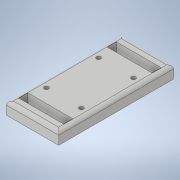
# Autodesk Inventor part: Tilt_Camera_Mount_Plate
Saved by Autodesk Inventor 2022 (Build 260153000, 153)
## iProperties
Created: 2020-01-01
Part Number: Tilt_Camera_Mount_Plate
Material: Generic
Document SubType Name: Modeling
Designer: KappaCat
Density: 1 g/cm^3
Appearance: Default
Author: KappaCat
Autodesk Inventor part; units mm, degrees
ref_plane "YZ Plane" through (0, 0, 0) normal (1, 0, 0) x (0, 1, 0)
ref_plane "XZ Plane" through (0, 0, 0) normal (0, 1, 0) x (-1, 0, 0)
ref_plane "XY Plane" through (0, 0, 0) normal (0, 0, 1) x (1, 0, 0)
sketch "Sketch1" plane through (0, 0, 0) normal (0, 1, 0) x (-1, 0, 0)
  line L0 (0, 0) -> (30, 0)
  line L1 (30, 0) -> (30, -65.85)
  line L2 (30, -65.85) -> (0, -65.85)
  line L3 (0, -65.85) -> (0, 0)
  dimension "d0" = 30
  dimension "d1" = 65.85
  constraints: 8 end point, 2 parallel, 1 horizontal, 1 perpendicular
  measures "d0" distance of L0.start L0.end
  measures "d1" distance of L0.end L1.end
extrude "Extrusion1" add sketch "Sketch1" along normal blind 7
sketch "Sketch2" plane through (0, 7, 0) normal (0, 1, 0) x (1, 0, 0)
  line L0 (-27.82, 5) -> (-2.18, 5)
  line L1 (-2.18, 5) -> (-2.18, 10.2)
  line L2 (-2.18, 10.2) -> (-27.82, 10.2)
  line L3 (-27.82, 10.2) -> (-27.82, 5)
  line L4 (-27.82, 55.65) -> (-2.18, 55.65)
  line L5 (-2.18, 55.65) -> (-2.18, 60.85)
  line L6 (-2.18, 60.85) -> (-27.82, 60.85)
  line L7 (-27.82, 60.85) -> (-27.82, 55.65)
  line L8 (-30, 0) -> (0, 0) projected
  line L9 (-15, 10.2) -> (-15, 55.65) construction
  line L10 (-30, 65.85) -> (-30, 0) construction
  line L11 (0, 65.85) -> (-30, 65.85) construction
  point P0 (-15, 5)
  point P1 (-15, 0)
  point P2 (-15, 32.925)
  point P3 (-30, 32.925)
  dimension "d4" = 25.64
  dimension "d5" = 5.2
  dimension "d6" = 5
  constraints: 18 end point, 6 midpoint, 4 parallel, 2 horizontal, 2 perpendicular, 2 point on line, 1 collinear, 1 horizontal alignment, 1 vertical alignment
  measures "d4" distance of L0.start L0.end
  measures "d5" distance of L2.end L0.start
  measures "d6" distance between parallel lines of L11 L6
extrude "Extrusion2" cut sketch "Sketch2" against normal up to next
sketch "Sketch3" plane through (0, 0, 0) normal (0, -1, 0) x (1, 0, 0)
  line L0 (-25, -47.85) -> (-5, -18) construction
  line L1 (-30, -65.85) -> (0, -65.85) construction
  line L2 (0, -65.85) -> (0, 0) construction
  point P0 (-25, -18)
  point P1 (-5, -47.85)
  point P2 (-15, -32.925)
  point P3 (-15, -65.85)
  point P4 (0, -32.925)
  dimension "d9" = 29.85
  dimension "d10" = 20
  constraints: 3 horizontal alignment, 3 midpoint, 3 vertical alignment, 2 end point
  measures "d9" distance of point (-25, -18) L0.start
  measures "d10" distance of point (-25, -18) L0.end
hole "Hole1" at (-25, 0, -47.85) at (-25, 0, -18) at (-5, 0, -18) at (-5, 0, -47.85) direction (0, 1, 0) diameter 2.46 end through all
fillet "Fillet1" radius 2 4 edges at (-30, 7, -32.925) (0, 7, -32.925) (-15, 7, -65.85) (-15, 7, 0)
body "Solid1"
